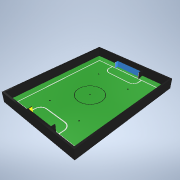
# Autodesk Inventor part: field
Saved by Autodesk Inventor 2020 (Build 240168000, 168)
## iProperties
Created: 2024-01-28
Part Number: field
Material: Типовые
Document SubType Name: Modeling
Designer: 4s
Density: 1 g/cm^3
Appearance: По умолчанию
Author: 4s
Autodesk Inventor part; units mm, degrees
ref_plane "YZ Plane" through (0, 0, 0) normal (1, 0, 0) x (0, 1, 0)
ref_plane "XZ Plane" through (0, 0, 0) normal (0, 1, 0) x (-1, 0, 0)
ref_plane "XY Plane" through (0, 0, 0) normal (0, 0, 1) x (1, 0, 0)
sketch "Эскиз1" plane through (0, 0, 0) normal (0, 1, 0) x (-1, 0, 0)
  line L0 (910, 1215) -> (-910, 1215)
  line L1 (-910, 1215) -> (-910, -1215)
  line L2 (-910, -1215) -> (910, -1215)
  line L3 (910, -1215) -> (910, 1215)
  line L4 (0, 0) -> (0, -1215) construction
  line L5 (0, 0) -> (910, 0) construction
  line L6 (950, 1255) -> (-950, 1255)
  line L7 (-950, 1255) -> (-950, -1255)
  line L8 (-950, -1255) -> (950, -1255)
  line L9 (950, -1255) -> (950, 1255)
  dimension "d0" = 2430
  dimension "d1" = 1820
  dimension "d2" = 40
  dimension "d3" = 40
  constraints: 20 end point, 4 horizontal, 4 parallel, 2 midpoint, 2 perpendicular, 2 vertical, 5 other
  measures "d0" distance of L2.end L0.start
  measures "d1" distance of L1.end L2.end
  measures "d2" distance between parallel lines of L0 L6
  measures "d3" distance between parallel lines of L3 L9
extrude "Выдавливание1" add sketch "Эскиз1" along normal blind 220
extrude "Выдавливание2" add sketch "Эскиз1" against normal blind 5 contours L3 L2 L1 L0 | L9 L8 L7 L6
sketch "Эскиз2" plane through (-910, 220, -1215) normal (0, 0, 1) x (1, 0, 0)
  line L0 (-40, -225) -> (-40, 0) construction
  line L1 (1860, 0) -> (-40, 0) construction
  line L2 (1860, 0) -> (1860, -225) construction
  line L3 (-40, -225) -> (1860, -225) construction
  line L4 (0, -220) -> (0, 0) construction
  line L5 (1860, 0) -> (-40, 0) construction
  line L6 (-40, 0) -> (1860, 0) construction
  line L7 (0, 0) -> (1820, 0) construction
  line L8 (1820, 0) -> (0, 0) construction
  line L9 (0, -220) -> (100, -220)
  line L10 (0, -220) -> (0, -200)
  line L11 (0, -200) -> (100, -220)
  line L12 (1820, -220) -> (1820, 0) construction
  line L13 (910, -220) -> (910, 0) construction
  line L14 (1820, -220) -> (1720, -220)
  line L15 (1820, -220) -> (1820, -200)
  line L16 (1820, -200) -> (1720, -220)
  point P0 (910, -220)
  dimension "d8" = 100
  dimension "d9" = 20
  constraints: 14 end point, 3 symmetric about line, 1 coincident, 1 horizontal, 1 midpoint, 1 point on line
  measures "d8" distance of L9.start L9.end
  measures "d9" distance of L9.start L10.end
extrude "Выдавливание3" add sketch "Эскиз2" along normal blind 2430
sketch "Эскиз3" plane through (-910, 220, 1215) normal (1, 0, 0) x (0, 0, -1)
  line L0 (2430, -200) -> (2430, 0) construction
  line L1 (0, -200) -> (0, 0) construction
  line L2 (0, -200) -> (2430, -200) construction
  line L3 (2430, -200) -> (2430, 0) construction
  line L4 (0, 0) -> (2430, 0) construction
  line L5 (0, -200) -> (0, 0) construction
  line L6 (1215, -220) -> (1215, 0) construction
  line L7 (2470, 0) -> (-40, 0) projected
  line L8 (0, -220) -> (100, -220)
  line L9 (100, -220) -> (0, -200)
  line L10 (0, -200) -> (0, -220)
  line L11 (2430, -220) -> (2330, -220)
  line L12 (2330, -220) -> (2430, -200)
  line L13 (2430, -200) -> (2430, -220)
  dimension "d14" = 100
  dimension "d15" = 20
  constraints: 14 end point, 3 symmetric about line, 1 horizontal, 1 midpoint, 1 perpendicular
  measures "d14" distance of L8.start L8.end
  measures "d15" distance of L2.start L8.start
extrude "Выдавливание4" add sketch "Эскиз3" along normal blind 1820
sketch "Эскиз4" plane through (0, 0, 0) normal (0, 1, 0) x (1, 0, 0)
  line L0 (-790, -1095) -> (790, -1095)
  line L1 (790, -1095) -> (790, 1095)
  line L2 (790, 1095) -> (-790, 1095)
  line L3 (-790, 1095) -> (-790, -1095)
  line L4 (0, 0) -> (0, 1215) construction
  line L5 (0, 0) -> (-910, 0) construction
  line L6 (810, -1115) -> (910, -1215) construction
  line L7 (-810, -1115) -> (810, -1115) construction
  line L8 (-910, -1215) -> (-810, -1115) construction
  line L9 (910, -1215) -> (-910, -1215) construction
  line L10 (-810, 1115) -> (-910, 1215) construction
  line L11 (-910, -1215) -> (-910, 1215) construction
  line L12 (-910, -1215) -> (-810, -1115) construction
  line L13 (-810, 1115) -> (-810, -1115) construction
  line L14 (910, 1215) -> (810, 1115) construction
  line L15 (-910, 1215) -> (910, 1215) construction
  line L16 (-810, 1115) -> (-910, 1215) construction
  line L17 (810, 1115) -> (-810, 1115) construction
  line L18 (910, 1215) -> (810, 1115) construction
  line L19 (810, -1115) -> (810, 1115) construction
  line L20 (810, -1115) -> (910, -1215) construction
  line L21 (910, 1215) -> (910, -1215) construction
  line L22 (810, 1115) -> (-810, 1115) construction
  line L23 (-810, 1115) -> (-810, -1115) construction
  line L24 (-810, -1115) -> (810, -1115) construction
  line L25 (810, -1115) -> (810, 1115) construction
  line L26 (-770, -1075) -> (770, -1075)
  line L27 (770, -1075) -> (770, 1075)
  line L28 (770, 1075) -> (-770, 1075)
  line L29 (-770, 1075) -> (-770, -1075)
  line L30 (-400, -1075) -> (400, -1075) construction
  line L31 (-400, -1075) -> (-400, -975)
  line L32 (-400, -825) -> (400, -825) construction
  line L33 (400, -825) -> (400, -1075) construction
  arc A0 (-400, -975) -> (-250, -825) centre (-250, -975) ccw construction
  arc A1 (-380, -975) -> (-250, -845) centre (-250, -975) ccw construction
  line L34 (-380, -975) -> (-380, -1075)
  line L35 (-250, -845) -> (0, -845)
  arc A2 (-250, -845) -> (-380, -975) centre (-250, -975) ccw
  arc A3 (-250, -825) -> (-400, -975) centre (-250, -975) ccw
  line L36 (-400, -975) -> (-400, -825) construction
  line L37 (-250, -825) -> (0, -825)
  line L38 (400, -1075) -> (400, -975)
  line L39 (380, -975) -> (380, -1075)
  line L40 (250, -845) -> (0, -845)
  arc A4 (380, -975) -> (250, -845) centre (250, -975) ccw
  arc A5 (400, -975) -> (250, -825) centre (250, -975) ccw
  line L41 (250, -825) -> (0, -825)
  line L42 (-400, 1075) -> (-400, 975)
  line L43 (-380, 975) -> (-380, 1075)
  line L44 (-250, 845) -> (0, 845)
  arc A6 (-380, 975) -> (-250, 845) centre (-250, 975) ccw
  arc A7 (-400, 975) -> (-250, 825) centre (-250, 975) ccw
  line L45 (-250, 825) -> (0, 825)
  line L46 (250, 845) -> (0, 845)
  line L47 (250, 825) -> (0, 825)
  arc A8 (250, 825) -> (400, 975) centre (250, 975) ccw
  arc A9 (250, 845) -> (380, 975) centre (250, 975) ccw
  line L48 (380, 975) -> (380, 1075)
  line L49 (400, 1075) -> (400, 975)
  point P0 (0, -1075)
  dimension "d18" = 120
  dimension "d19" = 120
  dimension "d20" = 20
  dimension "d21" = 20
  dimension "d22" = 800
  dimension "d23" = 250
  dimension "d24" = 300
  dimension "d25" = 20
  constraints: 56 end point, 26 symmetric about line, 20 point on circle, 10 centre point, 6 perpendicular, 5 tangent, 4 coincident, 4 horizontal, 4 parallel, 3 midpoint, 2 point on line, 2 vertical, 10 other
  measures "d18" distance between parallel lines of L11 L3
  measures "d19" distance between parallel lines of L15 L2
  measures "d20" distance between parallel lines of L2 L28
  measures "d21" distance between parallel lines of L3 L29
  measures "d22" distance of L30.start L30.end
  measures "d23" distance of L30.start L32.start
  measures "d24" diameter of A0
  measures "d25" radial gap between concentric circles of A0 A1
extrude "Выдавливание5" add sketch "Эскиз4" along normal blind 0.1 contours L3 L2 L1 L0 | L31 A3 L37 L41 A5 L38 L26 L39 A4 L40 L35 A2 L34 | L28 L43 A6 L44 L46 A9 L48 L49 A8 L47 L45 A7 L42
sketch "Эскиз5" plane through (0, 0, 0) normal (0, 1, 0) x (1, 0, 0)
  line L0 (0, 0) -> (-910, 0) construction
  line L1 (0, 0) -> (0, 1215) construction
  circle A0 centre (0, 0) radius 300
  circle A1 centre (0, 0) radius 290
  circle A2 centre (0, 0) radius 15
  line L2 (400, -975) -> (400, -1075) construction
  line L3 (400, -1075) -> (770, -1075) construction
  line L4 (770, -1075) -> (770, 1075) construction
  line L5 (770, 1075) -> (400, 1075) construction
  line L6 (400, 1075) -> (400, 975) construction
  arc A3 (250, 825) -> (400, 975) centre (250, 975) ccw construction
  line L7 (250, 825) -> (-250, 825) construction
  arc A4 (-400, 975) -> (-250, 825) centre (-250, 975) ccw construction
  line L8 (-400, 975) -> (-400, 1075) construction
  line L9 (-400, 1075) -> (-770, 1075) construction
  line L10 (-770, 1075) -> (-770, -1075) construction
  line L11 (-770, -1075) -> (-400, -1075) construction
  line L12 (-400, -1075) -> (-400, -975) construction
  arc A5 (-250, -825) -> (-400, -975) centre (-250, -975) ccw construction
  line L13 (-250, -825) -> (250, -825) construction
  arc A6 (400, -975) -> (250, -825) centre (250, -975) ccw construction
  line L14 (910, 1215) -> (810, 1115) construction
  line L15 (-910, 1215) -> (910, 1215) construction
  line L16 (-810, 1115) -> (-910, 1215) construction
  line L17 (810, 1115) -> (-810, 1115) construction
  line L18 (790, 1095) -> (-790, 1095) construction
  line L19 (-790, 1095) -> (-790, -1095) construction
  line L20 (-790, 1095) -> (790, 1095) construction
  line L21 (-790, 1095) -> (-390, 1095) construction
  line L22 (-390, 1095) -> (-390, 645) construction
  line L23 (-390, 645) -> (-790, 645) construction
  line L24 (-790, 645) -> (-790, 1095) construction
  circle A7 centre (-390, 645) radius 15
  circle A8 centre (-390, -645) radius 15
  circle A9 centre (390, 645) radius 15
  circle A10 centre (390, -645) radius 15
  dimension "d28" = 600
  dimension "d29" = 10
  dimension "d30" = 30
  dimension "d31" = 400
  dimension "d32" = 450
  dimension "d33" = 30
  constraints: 8 end point, 7 centre point, 4 coincident, 3 symmetric about line, 2 parallel, 1 horizontal, 1 perpendicular, 3 other
  measures "d28" diameter of A0
  measures "d29" radial gap between concentric circles of A0 A1
  measures "d30" diameter of A2
  measures "d31" distance of L22.end L23.end
  measures "d32" distance of L21.end L22.end
  measures "d33" diameter of A7
extrude "Выдавливание6" add sketch "Эскиз5" along normal blind 0.1
sketch "Эскиз6" plane through (0, 0, 0) normal (0, 1, 0) x (1, 0, 0)
  line L0 (-380, 1075) -> (-380, 975) construction
  arc A0 (-380, 975) -> (-250, 845) centre (-250, 975) ccw construction
  line L1 (-250, 845) -> (250, 845) construction
  arc A1 (250, 845) -> (380, 975) centre (250, 975) ccw construction
  line L2 (380, 975) -> (380, 1075) construction
  line L3 (380, 1075) -> (-380, 1075) construction
  line L4 (910, 1215) -> (810, 1115) construction
  line L5 (-910, 1215) -> (910, 1215) construction
  line L6 (-810, 1115) -> (-910, 1215) construction
  line L7 (810, 1115) -> (-810, 1115) construction
  line L8 (810, 1115) -> (-810, 1115) construction
  line L9 (-810, 1115) -> (-810, -1115) construction
  line L10 (-810, -1115) -> (810, -1115) construction
  line L11 (810, -1115) -> (810, 1115) construction
  line L12 (-790, -1095) -> (-790, 1095) construction
  line L13 (-790, 1095) -> (790, 1095) construction
  line L14 (790, 1095) -> (790, -1095) construction
  line L15 (790, -1095) -> (-790, -1095) construction
  line L16 (-790, -1095) -> (790, -1095) construction
  line L17 (790, -1095) -> (790, 1095) construction
  line L18 (790, 1095) -> (-790, 1095) construction
  line L19 (-790, 1095) -> (-790, -1095) construction
  arc A2 (400, -975) -> (250, -825) centre (250, -975) ccw construction
  line L20 (250, -825) -> (-250, -825) construction
  arc A3 (-250, -825) -> (-400, -975) centre (-250, -975) ccw construction
  line L21 (-400, -975) -> (-400, -1075) construction
  line L22 (-400, -1075) -> (-770, -1075) construction
  line L23 (-770, -1075) -> (-770, 1075) construction
  line L24 (-770, 1075) -> (-400, 1075) construction
  line L25 (-400, 1075) -> (-400, 975) construction
  arc A4 (-400, 975) -> (-250, 825) centre (-250, 975) ccw construction
  line L26 (-250, 825) -> (250, 825) construction
  arc A5 (250, 825) -> (400, 975) centre (250, 975) ccw construction
  line L27 (400, 975) -> (400, 1075) construction
  line L28 (400, 1075) -> (770, 1075) construction
  line L29 (770, 1075) -> (770, -1075) construction
  line L30 (770, -1075) -> (400, -1075) construction
  line L31 (400, -1075) -> (400, -975) construction
  line L32 (-380, 1075) -> (380, 1075) construction
  line L33 (380, 1075) -> (380, 975) construction
  arc A6 (250, 845) -> (380, 975) centre (250, 975) ccw construction
  line L34 (250, 845) -> (-250, 845) construction
  arc A7 (-380, 975) -> (-250, 845) centre (-250, 975) ccw construction
  line L35 (-380, 975) -> (-380, 1075) construction
  arc A8 (380, -975) -> (250, -845) centre (250, -975) ccw construction
  line L36 (380, -975) -> (380, -1075) construction
  line L37 (380, -1075) -> (-380, -1075) construction
  line L38 (-380, -1075) -> (-380, -975) construction
  arc A9 (-250, -845) -> (-380, -975) centre (-250, -975) ccw construction
  line L39 (-250, -845) -> (250, -845) construction
  line L40 (950, 1255) -> (-950, 1255) construction
  line L41 (-950, 1255) -> (-950, -1255) construction
  line L42 (-950, -1255) -> (950, -1255) construction
  line L43 (950, -1255) -> (950, 1255) construction
  line L44 (-910, -1215) -> (-910, 1215) construction
  line L45 (-910, 1215) -> (910, 1215) construction
  line L46 (910, 1215) -> (910, -1215) construction
  line L47 (910, -1215) -> (-910, -1215) construction
  line L48 (0, 0) -> (0, 1215) construction
  line L49 (400, -975) -> (400, -1075) construction
  line L50 (400, -1075) -> (770, -1075) construction
  line L51 (770, -1075) -> (770, 1075) construction
  line L52 (770, 1075) -> (400, 1075) construction
  line L53 (400, 1075) -> (400, 975) construction
  arc A10 (250, 825) -> (400, 975) centre (250, 975) ccw construction
  line L54 (250, 825) -> (-250, 825) construction
  arc A11 (-400, 975) -> (-250, 825) centre (-250, 975) ccw construction
  line L55 (-400, 975) -> (-400, 1075) construction
  line L56 (-400, 1075) -> (-770, 1075) construction
  line L57 (-770, 1075) -> (-770, -1075) construction
  line L58 (-770, -1075) -> (-400, -1075) construction
  line L59 (-400, -1075) -> (-400, -975) construction
  arc A12 (-250, -825) -> (-400, -975) centre (-250, -975) ccw construction
  line L60 (-250, -825) -> (250, -825) construction
  arc A13 (400, -975) -> (250, -825) centre (250, -975) ccw construction
  circle A14 centre (-390, -645) radius 15 construction
  circle A15 centre (390, 645) radius 15 construction
  circle A16 centre (390, -645) radius 15 construction
  circle A17 centre (-390, 645) radius 15 construction
  circle A18 centre (0, 0) radius 300 construction
  line L61 (0, 0) -> (-910, 0) construction
  line L62 (-910, 1215) -> (910, 1215) construction
  line L63 (-300, 1215) -> (300, 1215) construction
  line L64 (300, 1215) -> (300, 1149) construction
  line L65 (300, 1149) -> (-300, 1149)
  line L66 (-300, 1149) -> (-300, 1215) construction
  line L67 (-300, 1149) -> (-300, 1075)
  line L68 (380, 1075) -> (-380, 1075) construction
  line L69 (300, 1149) -> (300, 1075)
  line L70 (-300, 1164) -> (300, 1164)
  line L71 (-300, 1164) -> (-300, 1215)
  line L72 (300, 1164) -> (300, 1215)
  line L73 (-315, 1215) -> (-315, 1075)
  line L74 (-315, 1075) -> (-300, 1075)
  line L75 (-315, 1215) -> (-300, 1215)
  line L76 (315, 1215) -> (315, 1075)
  line L77 (300, 1075) -> (315, 1075)
  line L78 (300, 1215) -> (315, 1215)
  line L79 (300, -1149) -> (-300, -1149)
  line L80 (-300, -1149) -> (-300, -1075)
  line L81 (300, -1149) -> (300, -1075)
  line L82 (-300, -1164) -> (300, -1164)
  line L83 (-300, -1164) -> (-300, -1215)
  line L84 (300, -1164) -> (300, -1215)
  line L85 (-315, -1215) -> (-315, -1075)
  line L86 (-315, -1075) -> (-300, -1075)
  line L87 (-315, -1215) -> (-300, -1215)
  line L88 (315, -1215) -> (315, -1075)
  line L89 (300, -1075) -> (315, -1075)
  line L90 (300, -1215) -> (315, -1215)
  dimension "d36" = 600
  dimension "d38" = 74
  dimension "d39" = 15
  dimension "d40" = 15
  dimension "d41" = 15
  constraints: 54 end point, 12 symmetric about line, 9 point on line, 6 parallel, 5 perpendicular, 2 horizontal, 1 collinear, 1 vertical, 1 other
  measures "d36" distance of L64.end L65.end
  measures "d38" distance between parallel lines of L3 L65
  measures "d39" distance between parallel lines of L70 L65
  measures "d40" distance between parallel lines of L73 L66
  measures "d41" distance between parallel lines of L64 L76
extrude "Выдавливание7" add sketch "Эскиз6" along normal blind 150
